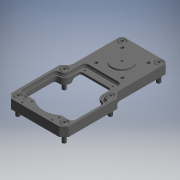
# Autodesk Inventor part: SLZ_63_Deckplatte#
Saved by Autodesk Inventor 2017.3 (Build 213256000, 256)
## iProperties
Part Number: SLZ_63_Deckplatte#
Material: Generic
Catalog Web Link: www.cadenas.de
Description: Deckplatte_SLZ63-Control-Tec
Vendor: ROSEKRIEGER
Document SubType Name: Modeling
Designer: partserver
Manufacturer: ROSEKRIEGER
Mass: 219.733 g
Surface Area: 785.713 cm^2
Volume: 219.733 cm^3
Density: 1 g/cm^3
Appearance: PSOLRGB-128-128-128
Category: PARTsolutions
Company: ROSEKRIEGER
Title: SLZ_63_Deckplatte#
Author: Cadenas PARTsolutions
Comments: Control-Tec
PSOL_IDENT_0: {$CADENAS_DATA\23d-libs\rose_krieger\linearkomponenten\pool_lineartechnik\_hubsaeule_zyliinder\elekt
PSOL_IDENT_1: rozylinder\elekzyl_slz63\parts\slz63_plfl_antrieb_deckplatte.prj},186 {VTYP=3D},{NB=SLZ_63_Deckplatt
PSOL_IDENT_2: e#},{LINA=SLZ_63_Deckplatte#},{NN=Deckplatte_SLZ63},{DATE=02.12.2020 11:16:23},{GEOMDATE=22.06.2016
PSOL_IDENT_3: 13:15:39},{VERSION=},{LINEID=10},{WBVAR=},{WBNUMERIC=}  {NB=SLZ_63_Deckplatte#},{LINA=SLZ_63_Deckpla
PSOL_IDENT_4: tte#},{KT=DUMMY},{IDNR=},{CODE=TQ3},{ARTIKEL=Elektrozylinder },{TYPE=SLZ 63 KG P PL},{BEST=SLZ_63_De
PSOL_IDENT_5: ckplatte},{VARIANTE=PL},{SPINDEL=KG 25x10},{SPINDELCODE=3.000},{SCHUTZARTVIS=IP54},{SCHUTZART=1},{HU
PSOL_IDENT_6: B1=0,[0:100]},{HINWEINBAUX=Hub + 288,5 mm},{DUMMYDURCH=10.000},{DUMMYLAENG=20.000},{HILFEHUB=105},{L
PSOL_IDENT_7: AENDOPPROFIL=184.500},{RF=1.000},{GRUNDKOE=288.500},{A=100},{B=80},{C=100},{D=125},{E=238},{F=40},{G=
PSOL_IDENT_8: M16x1.5},{H=104},{K=125},{L=105},{M=48},{N=56.5},{O=86},{P=18.5},{PPATH=sbl_lz70p_plfl.prj}
NB: SLZ_63_Deckplatte#
NN: Deckplatte_SLZ63
NT: Control-Tec
NBSYN: $BEST.#
LINA: SLZ_63_Deckplatte#
CATALOG: RK Rose+Krieger
ARTIKEL: Elektrozylinder
TYPE: SLZ 63 KG P PL
BEST: SLZ_63_Deckplatte
SPINDEL: KG 25x10
SPINDELCODE: 3
SCHUTZARTVIS: IP54
SCHUTZART: 1
HUB1: 0,[0:100]
HINWEINBAUX: Hub + 288,5 mm
DUMMYDURCH: 10
DUMMYLAENG: 20
HILFEHUB: 105
LAENDOPPROFIL: 184.5
RF: 1
GRUNDKOE: 288.5
A: 100
B: 80
C: 100
D: 125
E: 238
F: 40
G: M16x1.5
H: 104
K: 125
L: 105
M: 48
N: 56.5
O: 86
P: 18.5
SUPPLIER: ROSEKRIEGER
ARTICLENO: SLZ_63_Deckplatte#
BOMINFO: SLZ_63_Deckplatte#
CREATOR: CADENAS GmbH
Autodesk Inventor part; units mm, degrees
sketch "Sketch_2" plane through (0, 0, 0) normal (0, 0, 1) x (1, 0, 0)
  line L0 (-62.5, -178) -> (-52.5, -188)
  line L1 (-52.5, -188) -> (52.5, -188)
  line L2 (52.5, -188) -> (62.5, -178)
  line L3 (62.5, -178) -> (62.5, -72.5)
  line L4 (62.5, -72.5) -> (54.3934, -64.3934)
  arc A0 (50, -53.7868) -> (54.3934, -64.3934) centre (65, -53.7868) ccw
  line L5 (50, -53.7868) -> (50, 45)
  line L6 (50, 45) -> (45, 50)
  line L7 (45, 50) -> (-45, 50)
  line L8 (-45, 50) -> (-50, 45)
  line L9 (-50, 45) -> (-50, -53.7868)
  arc A1 (-54.3934, -64.3934) -> (-50, -53.7868) centre (-65, -53.7868) ccw
  line L10 (-54.3934, -64.3934) -> (-62.5, -72.5)
  line L11 (-62.5, -72.5) -> (-62.5, -178)
  circle A2 centre (30, -50.2) radius 2.1
  circle A3 centre (30, -166) radius 2.1
  circle A4 centre (-30, -50.2) radius 2.1
  circle A5 centre (-30, -166) radius 2.1
  arc A6 (-52.5, -154) -> (-46.5, -160) centre (-46.5, -154) ccw
  line L12 (-46.5, -160) -> (-30.3315, -160)
  arc A7 (-26.7631, -161.1765) -> (-30.3315, -160) centre (-30.3315, -166) ccw
  arc A8 (-26.7631, -161.1765) -> (26.7631, -161.1765) centre (0, -125) ccw
  arc A9 (30.3315, -160) -> (26.7631, -161.1765) centre (30.3315, -166) ccw
  line L13 (30.3315, -160) -> (46.5, -160)
  arc A10 (46.5, -160) -> (52.5, -154) centre (46.5, -154) ccw
  line L14 (52.5, -154) -> (52.5, -95.9437)
  arc A11 (52.5, -95.9437) -> (46.95, -89.9606) centre (46.5, -95.9437) ccw
  arc A12 (34, -76) -> (46.95, -89.9606) centre (48, -76) ccw
  line L15 (34, -76) -> (34, -62.2)
  arc A13 (34, -62.2) -> (28, -56.2) centre (28, -62.2) ccw
  line L16 (28, -56.2) -> (-28, -56.2)
  arc A14 (-28, -56.2) -> (-34, -62.2) centre (-28, -62.2) ccw
  line L17 (-34, -62.2) -> (-34, -76)
  arc A15 (-46.95, -89.9606) -> (-34, -76) centre (-48, -76) ccw
  arc A16 (-46.95, -89.9606) -> (-52.5, -95.9437) centre (-46.5, -95.9437) ccw
  line L18 (-52.5, -95.9437) -> (-52.5, -154)
  constraints: 38 end point, 26 point on circle, 17 centre point
extrude "Extrusion1" add sketch "Sketch_2" along normal blind 20
sketch "Sketch_1" plane through (0, 0, 19.8) normal (0, 0, 1) x (1, 0, 0)
  line L0 (-72.5, -198) -> (72.5, -198)
  line L1 (72.5, -198) -> (72.5, 60)
  line L2 (72.5, 60) -> (-72.5, 60)
  line L3 (-72.5, 60) -> (-72.5, -198)
  arc A0 (-58.8, -175.2248) -> (-57.9213, -177.3461) centre (-55.8, -175.2248) ccw
  line L4 (-57.9213, -177.3461) -> (-51.8461, -183.4213)
  arc A1 (-51.8461, -183.4213) -> (-49.7248, -184.3) centre (-49.7248, -181.3) ccw
  line L5 (-49.7248, -184.3) -> (49.7248, -184.3)
  arc A2 (49.7248, -184.3) -> (51.8461, -183.4213) centre (49.7248, -181.3) ccw
  line L6 (51.8461, -183.4213) -> (57.9213, -177.3461)
  arc A3 (57.9213, -177.3461) -> (58.8, -175.2248) centre (55.8, -175.2248) ccw
  line L7 (58.8, -175.2248) -> (58.8, -75.2752)
  arc A4 (58.8, -75.2752) -> (57.9213, -73.1539) centre (55.8, -75.2752) ccw
  line L8 (57.9213, -73.1539) -> (51.7771, -67.0097)
  arc A5 (46.3, -53.7868) -> (51.7771, -67.0097) centre (65, -53.7868) ccw
  line L9 (46.3, -53.7868) -> (46.3, 42.2248)
  arc A6 (46.3, 42.2248) -> (45.4213, 44.3461) centre (43.3, 42.2248) ccw
  line L10 (45.4213, 44.3461) -> (44.3461, 45.4213)
  arc A7 (44.3461, 45.4213) -> (42.2248, 46.3) centre (42.2248, 43.3) ccw
  line L11 (42.2248, 46.3) -> (-42.2248, 46.3)
  arc A8 (-42.2248, 46.3) -> (-44.3461, 45.4213) centre (-42.2248, 43.3) ccw
  line L12 (-44.3461, 45.4213) -> (-45.4213, 44.3461)
  arc A9 (-45.4213, 44.3461) -> (-46.3, 42.2248) centre (-43.3, 42.2248) ccw
  line L13 (-46.3, 42.2248) -> (-46.3, -53.7868)
  arc A10 (-51.7771, -67.0097) -> (-46.3, -53.7868) centre (-65, -53.7868) ccw
  line L14 (-51.7771, -67.0097) -> (-57.9213, -73.1539)
  arc A11 (-57.9213, -73.1539) -> (-58.8, -75.2752) centre (-55.8, -75.2752) ccw
  line L15 (-58.8, -75.2752) -> (-58.8, -175.2248)
  constraints: 32 end point, 24 point on circle, 12 centre point
extrude "Extrusion2" cut sketch "Sketch_1" along normal blind 0.2
sketch "Sketch_40" plane through (0, 0, 19.8) normal (0, 0, 1) x (1, 0, 0)
  arc A0 (-61, -175.2248) -> (-59.477, -178.9017) centre (-55.8, -175.2248) ccw
  line L0 (-59.477, -178.9017) -> (-53.4017, -184.977)
  arc A1 (-53.4017, -184.977) -> (-49.7248, -186.5) centre (-49.7248, -181.3) ccw
  line L1 (-49.7248, -186.5) -> (49.7248, -186.5)
  arc A2 (49.7248, -186.5) -> (53.4017, -184.977) centre (49.7248, -181.3) ccw
  line L2 (53.4017, -184.977) -> (59.477, -178.9017)
  arc A3 (59.477, -178.9017) -> (61, -175.2248) centre (55.8, -175.2248) ccw
  line L3 (61, -175.2248) -> (61, -75.2752)
  arc A4 (61, -75.2752) -> (59.477, -71.5983) centre (55.8, -75.2752) ccw
  line L4 (59.477, -71.5983) -> (53.3327, -65.4541)
  arc A5 (48.5, -53.7868) -> (53.3327, -65.4541) centre (65, -53.7868) ccw
  line L5 (48.5, -53.7868) -> (48.5, 42.2248)
  arc A6 (48.5, 42.2248) -> (46.977, 45.9017) centre (43.3, 42.2248) ccw
  line L6 (46.977, 45.9017) -> (45.9017, 46.977)
  arc A7 (45.9017, 46.977) -> (42.2248, 48.5) centre (42.2248, 43.3) ccw
  line L7 (42.2248, 48.5) -> (-42.2248, 48.5)
  arc A8 (-42.2248, 48.5) -> (-45.9017, 46.977) centre (-42.2248, 43.3) ccw
  line L8 (-45.9017, 46.977) -> (-46.977, 45.9017)
  arc A9 (-46.977, 45.9017) -> (-48.5, 42.2248) centre (-43.3, 42.2248) ccw
  line L9 (-48.5, 42.2248) -> (-48.5, -53.7868)
  arc A10 (-53.3327, -65.4541) -> (-48.5, -53.7868) centre (-65, -53.7868) ccw
  line L10 (-53.3327, -65.4541) -> (-59.477, -71.5983)
  arc A11 (-59.477, -71.5983) -> (-61, -75.2752) centre (-55.8, -75.2752) ccw
  line L11 (-61, -75.2752) -> (-61, -175.2248)
  arc A12 (-58.8, -175.2248) -> (-57.9213, -177.3461) centre (-55.8, -175.2248) ccw
  line L12 (-57.9213, -177.3461) -> (-51.8461, -183.4213)
  arc A13 (-51.8461, -183.4213) -> (-49.7248, -184.3) centre (-49.7248, -181.3) ccw
  line L13 (-49.7248, -184.3) -> (49.7248, -184.3)
  arc A14 (49.7248, -184.3) -> (51.8461, -183.4213) centre (49.7248, -181.3) ccw
  line L14 (51.8461, -183.4213) -> (57.9213, -177.3461)
  arc A15 (57.9213, -177.3461) -> (58.8, -175.2248) centre (55.8, -175.2248) ccw
  line L15 (58.8, -175.2248) -> (58.8, -75.2752)
  arc A16 (58.8, -75.2752) -> (57.9213, -73.1539) centre (55.8, -75.2752) ccw
  line L16 (57.9213, -73.1539) -> (51.7771, -67.0097)
  arc A17 (46.3, -53.7868) -> (51.7771, -67.0097) centre (65, -53.7868) ccw
  line L17 (46.3, -53.7868) -> (46.3, 42.2248)
  arc A18 (46.3, 42.2248) -> (45.4213, 44.3461) centre (43.3, 42.2248) ccw
  line L18 (45.4213, 44.3461) -> (44.3461, 45.4213)
  arc A19 (44.3461, 45.4213) -> (42.2248, 46.3) centre (42.2248, 43.3) ccw
  line L19 (42.2248, 46.3) -> (-42.2248, 46.3)
  arc A20 (-42.2248, 46.3) -> (-44.3461, 45.4213) centre (-42.2248, 43.3) ccw
  line L20 (-44.3461, 45.4213) -> (-45.4213, 44.3461)
  arc A21 (-45.4213, 44.3461) -> (-46.3, 42.2248) centre (-43.3, 42.2248) ccw
  line L21 (-46.3, 42.2248) -> (-46.3, -53.7868)
  arc A22 (-51.7771, -67.0097) -> (-46.3, -53.7868) centre (-65, -53.7868) ccw
  line L22 (-51.7771, -67.0097) -> (-57.9213, -73.1539)
  arc A23 (-57.9213, -73.1539) -> (-58.8, -75.2752) centre (-55.8, -75.2752) ccw
  line L23 (-58.8, -75.2752) -> (-58.8, -175.2248)
  constraints: 48 end point, 48 point on circle, 24 centre point
extrude "Extrusion3" cut sketch "Sketch_40" against normal blind 1.8
sketch "Sketch_3" plane through (0, 0, 10) normal (0, 0, 1) x (1, 0, 0)
  line L0 (-57.5, -93.6564) -> (-57.5, -157.0626)
  arc A0 (-57.5, -157.0626) -> (-51, -163.0417) centre (-51.5, -157.0626) ccw
  arc A1 (-38.1678, -173) -> (-51, -163.0417) centre (-50, -175) ccw
  arc A2 (-38.1678, -173) -> (-32.2518, -178) centre (-32.2518, -172) ccw
  line L1 (-32.2518, -178) -> (32.2518, -178)
  arc A3 (32.2518, -178) -> (38.1678, -173) centre (32.2518, -172) ccw
  arc A4 (51, -163.0417) -> (38.1678, -173) centre (50, -175) ccw
  arc A5 (51, -163.0417) -> (57.5, -157.0626) centre (51.5, -157.0626) ccw
  line L2 (57.5, -157.0626) -> (57.5, -93.6564)
  arc A6 (57.5, -93.6564) -> (50.3333, -87.771) centre (51.5, -93.6564) ccw
  arc A7 (38.625, -68.5094) -> (50.3333, -87.771) centre (48, -76) ccw
  arc A8 (38.625, -68.5094) -> (43, -56.025) centre (23, -56.025) ccw
  line L3 (43, -56.025) -> (43, -9.3274)
  arc A9 (43, -9.3274) -> (43, 9.3274) centre (0, 0) ccw
  line L4 (43, 9.3274) -> (43, 14.3229)
  arc A10 (43, 14.3229) -> (31.5419, 21.5369) centre (35, 14.3229) ccw
  arc A11 (21.5369, 31.5419) -> (31.5419, 21.5369) centre (28.3, 28.3) ccw
  arc A12 (21.5369, 31.5419) -> (14.3229, 43) centre (14.3229, 35) ccw
  line L5 (14.3229, 43) -> (9.3274, 43)
  arc A13 (9.3274, 43) -> (-9.3274, 43) centre (0, 0) ccw
  line L6 (-9.3274, 43) -> (-14.3229, 43)
  arc A14 (-14.3229, 43) -> (-21.5369, 31.5419) centre (-14.3229, 35) ccw
  arc A15 (-31.5419, 21.5369) -> (-21.5369, 31.5419) centre (-28.3, 28.3) ccw
  arc A16 (-31.5419, 21.5369) -> (-43, 14.3229) centre (-35, 14.3229) ccw
  line L7 (-43, 14.3229) -> (-43, 9.3274)
  arc A17 (-43, 9.3274) -> (-43, -9.3274) centre (0, 0) ccw
  line L8 (-43, -9.3274) -> (-43, -56.025)
  arc A18 (-43, -56.025) -> (-38.625, -68.5094) centre (-23, -56.025) ccw
  arc A19 (-50.3333, -87.771) -> (-38.625, -68.5094) centre (-48, -76) ccw
  arc A20 (-50.3333, -87.771) -> (-57.5, -93.6564) centre (-51.5, -93.6564) ccw
  constraints: 42 point on circle, 21 centre point, 18 end point
extrude "Extrusion4" cut sketch "Sketch_3" along normal blind 10
sketch "Sketch_8" plane through (0, 0, 10) normal (0, 0, 1) x (1, 0, 0)
  circle A0 centre (28.3, -28.3) radius 7.5
  constraints: 1 centre point
extrude "Extrusion5" add sketch "Sketch_8" along normal blind 9.5
sketch "Sketch_9" plane through (0, 0, 10) normal (0, 0, 1) x (1, 0, 0)
  circle A0 centre (-28.3, -28.3) radius 7.5
  constraints: 1 centre point
extrude "Extrusion6" add sketch "Sketch_9" along normal blind 9.5
sketch "Sketch_5" plane through (0, 0, 19.5) normal (0, 0, 1) x (1, 0, 0)
  circle A0 centre (0, 0) radius 44
  constraints: 1 centre point
extrude "Extrusion7" cut sketch "Sketch_5" along normal blind 0.5
sketch "Sketch_4" plane through (0, 0, 0) normal (0, 0, 1) x (1, 0, 0)
  line L0 (-57.5, -92.9931) -> (-57.5, -157.0069)
  arc A0 (-57.5, -157.0069) -> (-49.7222, -165.0039) centre (-49.5, -157.0069) ccw
  arc A1 (-40.3935, -172.2222) -> (-49.7222, -165.0039) centre (-50, -175) ccw
  arc A2 (-40.3935, -172.2222) -> (-32.7084, -178) centre (-32.7084, -170) ccw
  line L1 (-32.7084, -178) -> (32.7084, -178)
  arc A3 (32.7084, -178) -> (40.3935, -172.2222) centre (32.7084, -170) ccw
  arc A4 (49.7222, -165.0039) -> (40.3935, -172.2222) centre (50, -175) ccw
  arc A5 (49.7222, -165.0039) -> (57.5, -157.0069) centre (49.5, -157.0069) ccw
  line L2 (57.5, -157.0069) -> (57.5, -92.9931)
  arc A6 (57.5, -92.9931) -> (49.7222, -84.9961) centre (49.5, -92.9931) ccw
  arc A7 (40, -75) -> (49.7222, -84.9961) centre (50, -75) ccw
  line L3 (40, -75) -> (40, -48)
  arc A8 (40, -48) -> (32, -40) centre (32, -48) ccw
  line L4 (32, -40) -> (-32, -40)
  arc A9 (-32, -40) -> (-40, -48) centre (-32, -48) ccw
  line L5 (-40, -48) -> (-40, -75)
  arc A10 (-49.7222, -84.9961) -> (-40, -75) centre (-50, -75) ccw
  arc A11 (-49.7222, -84.9961) -> (-57.5, -92.9931) centre (-49.5, -92.9931) ccw
  constraints: 24 point on circle, 12 centre point, 12 end point
extrude "Extrusion8" cut sketch "Sketch_4" along normal blind 5
sketch "Sketch_41" plane through (0, 0, 5) normal (0, 0, 1) x (1, 0, 0)
  line L0 (-56.5, -92.9931) -> (-56.5, -157.0069)
  arc A0 (-56.5, -157.0069) -> (-49.6944, -164.0042) centre (-49.5, -157.0069) ccw
  arc A1 (-39.4329, -171.9444) -> (-49.6944, -164.0042) centre (-50, -175) ccw
  arc A2 (-39.4329, -171.9444) -> (-32.7084, -177) centre (-32.7084, -170) ccw
  line L1 (-32.7084, -177) -> (32.7084, -177)
  arc A3 (32.7084, -177) -> (39.4329, -171.9444) centre (32.7084, -170) ccw
  arc A4 (49.6944, -164.0042) -> (39.4329, -171.9444) centre (50, -175) ccw
  arc A5 (49.6944, -164.0042) -> (56.5, -157.0069) centre (49.5, -157.0069) ccw
  line L2 (56.5, -157.0069) -> (56.5, -92.9931)
  arc A6 (56.5, -92.9931) -> (49.6944, -85.9958) centre (49.5, -92.9931) ccw
  arc A7 (39, -75) -> (49.6944, -85.9958) centre (50, -75) ccw
  line L3 (39, -75) -> (39, -48)
  arc A8 (39, -48) -> (32, -41) centre (32, -48) ccw
  line L4 (32, -41) -> (-32, -41)
  arc A9 (-32, -41) -> (-39, -48) centre (-32, -48) ccw
  line L5 (-39, -48) -> (-39, -75)
  arc A10 (-49.6944, -85.9958) -> (-39, -75) centre (-50, -75) ccw
  arc A11 (-49.6944, -85.9958) -> (-56.5, -92.9931) centre (-49.5, -92.9931) ccw
  line L6 (-54.3, -92.9931) -> (-54.3, -157.0069)
  arc A12 (-54.3, -157.0069) -> (-49.6333, -161.8051) centre (-49.5, -157.0069) ccw
  arc A13 (-37.3195, -171.3333) -> (-49.6333, -161.8051) centre (-50, -175) ccw
  arc A14 (-37.3195, -171.3333) -> (-32.7084, -174.8) centre (-32.7084, -170) ccw
  line L7 (-32.7084, -174.8) -> (32.7084, -174.8)
  arc A15 (32.7084, -174.8) -> (37.3195, -171.3333) centre (32.7084, -170) ccw
  arc A16 (49.6333, -161.8051) -> (37.3195, -171.3333) centre (50, -175) ccw
  arc A17 (49.6333, -161.8051) -> (54.3, -157.0069) centre (49.5, -157.0069) ccw
  line L8 (54.3, -157.0069) -> (54.3, -92.9931)
  arc A18 (54.3, -92.9931) -> (49.6333, -88.1949) centre (49.5, -92.9931) ccw
  arc A19 (36.8, -75) -> (49.6333, -88.1949) centre (50, -75) ccw
  line L9 (36.8, -75) -> (36.8, -48)
  arc A20 (36.8, -48) -> (32, -43.2) centre (32, -48) ccw
  line L10 (32, -43.2) -> (-32, -43.2)
  arc A21 (-32, -43.2) -> (-36.8, -48) centre (-32, -48) ccw
  line L11 (-36.8, -48) -> (-36.8, -75)
  arc A22 (-49.6333, -88.1949) -> (-36.8, -75) centre (-50, -75) ccw
  arc A23 (-49.6333, -88.1949) -> (-54.3, -92.9931) centre (-49.5, -92.9931) ccw
  constraints: 48 point on circle, 24 centre point, 24 end point
extrude "Extrusion9" cut sketch "Sketch_41" along normal blind 2
sketch "Sketch_6" plane through (0, 0, 0) normal (1, 0, 0) x (0, 0, -1)
  line L0 (3, 0) -> (-19, 0)
  line L1 (-19, 0) -> (-19, 14)
  line L2 (-19, 14) -> (0, 14)
  line L3 (0, 14) -> (0, 22.4)
  line L4 (0, 22.4) -> (3, 22.4)
  line L5 (3, 22.4) -> (3, 0)
  line L6 (3, 0) -> (-19, 0)
  constraints: 14 end point
revolve "Revolution1" add sketch "Sketch_6" angle 360 about axis through (0, 0, -3) along (0, 0, -1)
sketch "Sketch_7" plane through (0, 0, 0) normal (1, 0, 0) x (0, 0, -1)
  line L0 (3, 0) -> (-19, 0)
  line L1 (-19, 0) -> (-19, 8.5)
  line L2 (-19, 8.5) -> (-18.5, 8)
  line L3 (-18.5, 8) -> (-17.625, 8)
  line L4 (-17.625, 8) -> (-17.625, 8.25)
  line L5 (-17.625, 8.25) -> (-16.225, 8.25)
  line L6 (-16.225, 8.25) -> (-16.225, 8)
  line L7 (-16.225, 8) -> (-5.8, 8)
  line L8 (-5.8, 8) -> (-5.8, 7)
  line L9 (-5.8, 7) -> (-3.3, 7)
  line L10 (-3.3, 7) -> (-3.3, 2.5)
  line L11 (-3.3, 2.5) -> (3, 2.5)
  line L12 (3, 2.5) -> (3, 0)
  line L13 (3, 0) -> (-19, 0)
  constraints: 28 end point
revolve "Revolution2" cut sketch "Sketch_7" angle 360 about axis through (0, 0, -3) along (0, 0, -1)
sketch "Sketch_10" plane through (28.25, 0, 0) normal (1, 0, 0) x (0, 0, -1)
  line L0 (0, 28.25) -> (-19.1429, 28.25)
  line L1 (-19.1429, 28.25) -> (-17.1, 31.65)
  line L2 (-17.1, 31.65) -> (-15.9, 31.65)
  line L3 (-15.9, 31.65) -> (-15.9, 32.455)
  line L4 (-15.9, 32.455) -> (-14.2, 32.455)
  line L5 (-14.2, 32.455) -> (-14.2, 31.65)
  line L6 (-14.2, 31.65) -> (-0.75, 31.65)
  line L7 (-0.75, 31.65) -> (0, 32.4)
  line L8 (0, 32.4) -> (0, 28.25)
  line L9 (0, 28.25) -> (-19.1429, 28.25)
  constraints: 20 end point
revolve "Revolution3" cut sketch "Sketch_10" angle 360 about axis through (28.25, 28.25, 0) along (0, 0, -1)
pattern_linear "Rectangular Pattern1" count 2 spacing 56.5 along (-1, 0, 0) count 2 spacing 56.5 along (0, -1, 0) of "Revolution3"
sketch "Sketch_12" plane through (40, 0, 0) normal (1, 0, 0) x (0, 0, -1)
  line L0 (0, 40) -> (-20, 40)
  line L1 (-20, 40) -> (-20, 44.5)
  line L2 (-20, 44.5) -> (-8.6, 44.5)
  line L3 (-8.6, 44.5) -> (-8.6, 44.25)
  line L4 (-8.6, 44.25) -> (-7.6, 44.25)
  line L5 (-7.6, 44.25) -> (-7.6, 46.7)
  line L6 (-7.6, 46.7) -> (-8.6, 46.7)
  line L7 (-8.6, 46.7) -> (-8.6, 47.5)
  line L8 (-8.6, 47.5) -> (0, 47.5)
  line L9 (0, 47.5) -> (0, 40)
  line L10 (0, 40) -> (-20, 40)
  constraints: 22 end point
revolve "Revolution4" cut sketch "Sketch_12" angle 360 about axis through (40, 40, 0) along (0, 0, -1)
sketch "Sketch_13" plane through (-40, 0, 0) normal (1, 0, 0) x (0, 0, -1)
  line L0 (0, 40) -> (-20, 40)
  line L1 (-20, 40) -> (-20, 44.5)
  line L2 (-20, 44.5) -> (-8.6, 44.5)
  line L3 (-8.6, 44.5) -> (-8.6, 44.25)
  line L4 (-8.6, 44.25) -> (-7.6, 44.25)
  line L5 (-7.6, 44.25) -> (-7.6, 46.7)
  line L6 (-7.6, 46.7) -> (-8.6, 46.7)
  line L7 (-8.6, 46.7) -> (-8.6, 47.5)
  line L8 (-8.6, 47.5) -> (0, 47.5)
  line L9 (0, 47.5) -> (0, 40)
  line L10 (0, 40) -> (-20, 40)
  constraints: 22 end point
revolve "Revolution5" cut sketch "Sketch_13" angle 360 about axis through (-40, 40, 0) along (0, 0, -1)
sketch "Sketch_14" plane through (50, 0, 0) normal (1, 0, 0) x (0, 0, -1)
  line L0 (0, -75) -> (-20, -75)
  line L1 (-20, -75) -> (-20, -70.5)
  line L2 (-20, -70.5) -> (-8.6, -70.5)
  line L3 (-8.6, -70.5) -> (-8.6, -70.75)
  line L4 (-8.6, -70.75) -> (-7.6, -70.75)
  line L5 (-7.6, -70.75) -> (-7.6, -68.3)
  line L6 (-7.6, -68.3) -> (-8.6, -68.3)
  line L7 (-8.6, -68.3) -> (-8.6, -67.5)
  line L8 (-8.6, -67.5) -> (0, -67.5)
  line L9 (0, -67.5) -> (0, -75)
  line L10 (0, -75) -> (-20, -75)
  constraints: 22 end point
revolve "Revolution6" cut sketch "Sketch_14" angle 360 about axis through (50, -75, 0) along (0, 0, -1)
pattern_linear "Rectangular Pattern2" count 2 spacing 100 along (-1, 0, 0) count 2 spacing 100 along (0, -1, 0) of "Revolution6"
sketch "Sketch_16" plane through (40, 0, 0) normal (1, 0, 0) x (0, 0, -1)
  line L0 (0.4, 40) -> (-37.6, 40)
  line L1 (-37.6, 40) -> (-37.6, 43.233)
  line L2 (-37.6, 43.233) -> (-36.833, 44)
  line L3 (-36.833, 44) -> (-8, 44)
  arc A0 (-8, 44) -> (-7.6, 44.4) centre (-8, 44.4) ccw
  line L4 (-7.6, 44.4) -> (-7.6, 46.1)
  arc A1 (-7.2, 46.5) -> (-7.6, 46.1) centre (-7.2, 46.1) ccw
  line L5 (-7.2, 46.5) -> (-0.4, 46.5)
  line L6 (-0.4, 46.5) -> (0.4, 45.7)
  line L7 (0.4, 45.7) -> (0.4, 40)
  line L8 (0.4, 40) -> (-37.6, 40)
  constraints: 18 end point, 4 point on circle, 2 centre point
revolve "Revolution7" add sketch "Sketch_16" angle 360 about axis through (40, 40, -0.4) along (0, 0, -1)
thread "Thread1" size "M8x1.25" class "6g" standard "ISO Metric profile" full length
sketch "Sketch_17" plane through (-40, 0, 0) normal (1, 0, 0) x (0, 0, -1)
  line L0 (0.4, 40) -> (-37.6, 40)
  line L1 (-37.6, 40) -> (-37.6, 43.233)
  line L2 (-37.6, 43.233) -> (-36.833, 44)
  line L3 (-36.833, 44) -> (-8, 44)
  arc A0 (-8, 44) -> (-7.6, 44.4) centre (-8, 44.4) ccw
  line L4 (-7.6, 44.4) -> (-7.6, 46.1)
  arc A1 (-7.2, 46.5) -> (-7.6, 46.1) centre (-7.2, 46.1) ccw
  line L5 (-7.2, 46.5) -> (-0.4, 46.5)
  line L6 (-0.4, 46.5) -> (0.4, 45.7)
  line L7 (0.4, 45.7) -> (0.4, 40)
  line L8 (0.4, 40) -> (-37.6, 40)
  constraints: 18 end point, 4 point on circle, 2 centre point
revolve "Revolution8" add sketch "Sketch_17" angle 360 about axis through (-40, 40, -0.4) along (0, 0, -1)
thread "Thread2" size "M8x1.25" class "6g" standard "ISO Metric profile" full length
sketch "Sketch_18" plane through (50, 0, 0) normal (1, 0, 0) x (0, 0, -1)
  line L0 (0.4, -75) -> (-37.6, -75)
  line L1 (-37.6, -75) -> (-37.6, -71.767)
  line L2 (-37.6, -71.767) -> (-36.833, -71)
  line L3 (-36.833, -71) -> (-8, -71)
  arc A0 (-8, -71) -> (-7.6, -70.6) centre (-8, -70.6) ccw
  line L4 (-7.6, -70.6) -> (-7.6, -68.9)
  arc A1 (-7.2, -68.5) -> (-7.6, -68.9) centre (-7.2, -68.9) ccw
  line L5 (-7.2, -68.5) -> (-0.4, -68.5)
  line L6 (-0.4, -68.5) -> (0.4, -69.3)
  line L7 (0.4, -69.3) -> (0.4, -75)
  line L8 (0.4, -75) -> (-37.6, -75)
  constraints: 18 end point, 4 point on circle, 2 centre point
revolve "Revolution9" add sketch "Sketch_18" angle 360 about axis through (50, -75, -0.4) along (0, 0, -1)
thread "Thread3" size "M8x1.25" class "6g" standard "ISO Metric profile" full length
pattern_linear "Rectangular Pattern3" count 2 spacing 100 along (-1, 0, 0) count 2 spacing 100 along (0, -1, 0) of "Revolution9"
sketch "Sketch_20" plane through (0, 0, -0.4) normal (0, 0, 1) x (1, 0, 0)
  line L0 (-43, 38.2679) -> (-40, 36.5359)
  line L1 (-40, 36.5359) -> (-37, 38.2679)
  line L2 (-37, 38.2679) -> (-37, 41.7321)
  line L3 (-37, 41.7321) -> (-40, 43.4641)
  line L4 (-40, 43.4641) -> (-43, 41.7321)
  line L5 (-43, 41.7321) -> (-43, 38.2679)
  constraints: 12 end point
extrude "Extrusion10" cut sketch "Sketch_20" along normal blind 4
sketch "Sketch_21" plane through (0, 0, -0.4) normal (0, 0, 1) x (1, 0, 0)
  line L0 (37, 38.2679) -> (40, 36.5359)
  line L1 (40, 36.5359) -> (43, 38.2679)
  line L2 (43, 38.2679) -> (43, 41.7321)
  line L3 (43, 41.7321) -> (40, 43.4641)
  line L4 (40, 43.4641) -> (37, 41.7321)
  line L5 (37, 41.7321) -> (37, 38.2679)
  constraints: 12 end point
extrude "Extrusion11" cut sketch "Sketch_21" along normal blind 4
sketch "Sketch_22" plane through (0, 0, -0.4) normal (0, 0, 1) x (1, 0, 0)
  line L0 (47, -76.7321) -> (50, -78.4641)
  line L1 (50, -78.4641) -> (53, -76.7321)
  line L2 (53, -76.7321) -> (53, -73.2679)
  line L3 (53, -73.2679) -> (50, -71.5359)
  line L4 (50, -71.5359) -> (47, -73.2679)
  line L5 (47, -73.2679) -> (47, -76.7321)
  constraints: 12 end point
extrude "Extrusion12" cut sketch "Sketch_22" along normal blind 4
pattern_linear "Rectangular Pattern4" count 2 spacing 100 along (-1, 0, 0) count 2 spacing 100 along (0, -1, 0) of "Extrusion12"
sketch "Sketch_24" plane through (32.5, 0, 0) normal (1, 0, 0) x (0, 0, -1)
  line L0 (3, -183) -> (0, -183)
  line L1 (0, -183) -> (0, -181)
  line L2 (0, -181) -> (2.5, -181)
  line L3 (2.5, -181) -> (3, -181.5)
  line L4 (3, -181.5) -> (3, -183)
  line L5 (3, -183) -> (0, -183)
  constraints: 12 end point
revolve "Revolution10" add sketch "Sketch_24" angle 360 about axis through (32.5, -183, -3) along (0, 0, -1)
sketch "Sketch_25" plane through (-32.5, 0, 0) normal (1, 0, 0) x (0, 0, -1)
  line L0 (3, -183) -> (0, -183)
  line L1 (0, -183) -> (0, -181)
  line L2 (0, -181) -> (2.5, -181)
  line L3 (2.5, -181) -> (3, -181.5)
  line L4 (3, -181.5) -> (3, -183)
  line L5 (3, -183) -> (0, -183)
  constraints: 12 end point
revolve "Revolution11" add sketch "Sketch_25" angle 360 about axis through (-32.5, -183, -3) along (0, 0, -1)
ref_plane "ANTRIEBABDECKUNG_XY" through (0, 0, 0) normal (0, 0, 1) x (1, 0, 0)
ref_plane "ANTRIEBABDECKUNG_YZ" through (0, 0, 0) normal (1, 0, 0) x (0, 1, 0)
ref_plane "ANTRIEBABDECKUNG_ZX" through (0, 0, 0) normal (0, 1, 0) x (0, 0, 1)
ref_plane "ANTRIEBDECKPLATTE_XY" through (0, 0, 20) normal (0, 0, -1) x (1, 0, 0)
ref_plane "ANTRIEBDECKPLATTE_YZ" through (0, 0, 20) normal (1, 0, 0) x (0, -1, 0)
ref_plane "ANTRIEBDECKPLATTE_ZX" through (0, 0, 20) normal (0, -1, 0) x (0, 0, -1)
ref_plane "DP31_XY" through (0, -183, -3) normal (1, 0, 0) x (0, 0, -1)
ref_plane "DP31_YZ" through (0, -183, -3) normal (0, 0, -1) x (0, 1, 0)
ref_plane "DP31_ZX" through (0, -183, -3) normal (0, 1, 0) x (1, 0, 0)
ref_plane "DP32_XY" through (0, -183, 0) normal (1, 0, 0) x (0, 0, -1)
ref_plane "DP32_YZ" through (0, -183, 0) normal (0, 0, -1) x (0, 1, 0)
ref_plane "DP32_ZX" through (0, -183, 0) normal (0, 1, 0) x (1, 0, 0)
ref_plane "DP451_XY" through (0, 22.5, -3) normal (1, 0, 0) x (0, 0, -1)
ref_plane "DP451_YZ" through (0, 22.5, -3) normal (0, 0, -1) x (0, 1, 0)
ref_plane "DP451_ZX" through (0, 22.5, -3) normal (0, 1, 0) x (1, 0, 0)
ref_plane "DP452_XY" through (0, -22.5, -3) normal (1, 0, 0) x (0, 0, -1)
ref_plane "DP452_YZ" through (0, -22.5, -3) normal (0, 0, -1) x (0, 1, 0)
ref_plane "DP452_ZX" through (0, -22.5, -3) normal (0, 1, 0) x (1, 0, 0)
ref_plane "DPA1_XY" through (45, 50, 0) normal (0, 0, 1) x (1, 0, 0)
ref_plane "DPA1_YZ" through (45, 50, 0) normal (1, 0, 0) x (0, 1, 0)
ref_plane "DPA1_ZX" through (45, 50, 0) normal (0, 1, 0) x (0, 0, 1)
ref_plane "DPA2_XY" through (45, -50, 0) normal (0, 0, 1) x (1, 0, 0)
ref_plane "DPA2_YZ" through (45, -50, 0) normal (1, 0, 0) x (0, 1, 0)
ref_plane "DPA2_ZX" through (45, -50, 0) normal (0, 1, 0) x (0, 0, 1)
ref_plane "DPC1_XY" through (50, 45, 0) normal (0, 0, 1) x (1, 0, 0)
ref_plane "DPC1_YZ" through (50, 45, 0) normal (1, 0, 0) x (0, 1, 0)
ref_plane "DPC1_ZX" through (50, 45, 0) normal (0, 1, 0) x (0, 0, 1)
ref_plane "DPC2_XY" through (-50, 45, 0) normal (0, 0, 1) x (1, 0, 0)
ref_plane "DPC2_YZ" through (-50, 45, 0) normal (1, 0, 0) x (0, 1, 0)
ref_plane "DPC2_ZX" through (-50, 45, 0) normal (0, 1, 0) x (0, 0, 1)
ref_plane "DPD1_XY" through (62.5, -178, 0) normal (0, 0, 1) x (1, 0, 0)
ref_plane "DPD1_YZ" through (62.5, -178, 0) normal (1, 0, 0) x (0, 1, 0)
ref_plane "DPD1_ZX" through (62.5, -178, 0) normal (0, 1, 0) x (0, 0, 1)
ref_plane "DPD2_XY" through (-62.5, -178, 0) normal (0, 0, 1) x (1, 0, 0)
ref_plane "DPD2_YZ" through (-62.5, -178, 0) normal (1, 0, 0) x (0, 1, 0)
ref_plane "DPD2_ZX" through (-62.5, -178, 0) normal (0, 1, 0) x (0, 0, 1)
ref_plane "DPE1_XY" through (-45, 50, 0) normal (0, 0, 1) x (1, 0, 0)
ref_plane "DPE1_YZ" through (-45, 50, 0) normal (1, 0, 0) x (0, 1, 0)
ref_plane "DPE1_ZX" through (-45, 50, 0) normal (0, 1, 0) x (0, 0, 1)
ref_plane "DPE2_XY" through (-52.5, -188, 0) normal (0, 0, 1) x (1, 0, 0)
ref_plane "DPE2_YZ" through (-52.5, -188, 0) normal (1, 0, 0) x (0, 1, 0)
ref_plane "DPE2_ZX" through (-52.5, -188, 0) normal (0, 1, 0) x (0, 0, 1)
ref_plane "DPH2_XY" through (0, 50, 0) normal (1, 0, 0) x (0, 0, -1)
ref_plane "DPH2_YZ" through (0, 50, 0) normal (0, 0, -1) x (0, 1, 0)
ref_plane "DPH2_ZX" through (0, 50, 0) normal (0, 1, 0) x (1, 0, 0)
ref_plane "DPK1_XY" through (0, 0, 0) normal (0, 0, 1) x (1, 0, 0)
ref_plane "DPK1_YZ" through (0, 0, 0) normal (1, 0, 0) x (0, 1, 0)
ref_plane "DPK1_ZX" through (0, 0, 0) normal (0, 1, 0) x (0, 0, 1)
ref_plane "DPK2_XY" through (0, -125, 0) normal (0, 0, 1) x (1, 0, 0)
ref_plane "DPK2_YZ" through (0, -125, 0) normal (1, 0, 0) x (0, 1, 0)
ref_plane "DPK2_ZX" through (0, -125, 0) normal (0, 1, 0) x (0, 0, 1)
ref_plane "DPN1_XY" through (28.25, 28.25, 0) normal (0, 0, 1) x (1, 0, 0)
ref_plane "DPN1_YZ" through (28.25, 28.25, 0) normal (1, 0, 0) x (0, 1, 0)
ref_plane "DPN1_ZX" through (28.25, 28.25, 0) normal (0, 1, 0) x (0, 0, 1)
ref_plane "DPN2_XY" through (-28.25, 28.25, 0) normal (0, 0, 1) x (1, 0, 0)
ref_plane "DPN2_YZ" through (-28.25, 28.25, 0) normal (1, 0, 0) x (0, 1, 0)
ref_plane "DPN2_ZX" through (-28.25, 28.25, 0) normal (0, 1, 0) x (0, 0, 1)
ref_plane "DPNULL1_XY" through (0, -183, -3) normal (1, 0, 0) x (0, 0, -1)
ref_plane "DPNULL1_YZ" through (0, -183, -3) normal (0, 0, -1) x (0, 1, 0)
ref_plane "DPNULL1_ZX" through (0, -183, -3) normal (0, 1, 0) x (1, 0, 0)
ref_plane "DPO2_XY" through (0, 50, 0) normal (1, 0, 0) x (0, 0, -1)
ref_plane "DPO2_YZ" through (0, 50, 0) normal (0, 0, -1) x (0, 1, 0)
ref_plane "DPO2_ZX" through (0, 50, 0) normal (0, 1, 0) x (1, 0, 0)
ref_plane "DPX1_XY" through (0, -183, -3) normal (1, 0, 0) x (0, 0, -1)
ref_plane "DPX1_YZ" through (0, -183, -3) normal (0, 0, -1) x (0, 1, 0)
ref_plane "DPX1_ZX" through (0, -183, -3) normal (0, 1, 0) x (1, 0, 0)
body "Solid1"
